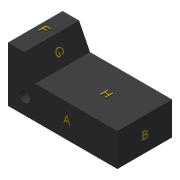
# Autodesk Inventor part: Component_1
Saved by Autodesk Inventor 2022 Beta2 (Build 260130000, 130) ContinuousBuild 0
## iProperties
Shininess: 64.0
Length Units: 11269
Angle Units: 11279
Time Units: 11290
Mass Units: 11283
Length Display Precision: 3
Angle Display Precision: 2
Compacted: True
Part Number: Component_1
Document SubType Name: Modeling
Created: 2004-04-20
Designer: mpaknia
Manufacturer: Standard
Standards Organization: Custom
Density: 1 g/cm^3
Material: Generic
Appearance: Generic
Density: 0.0
Volumn: 0.0
Area: 0.0
PropertySet Name: Model Information
Control State: 0
Master: False
Checked Out: False
Author: mpaknia
Autodesk Inventor part; units mm, degrees
note: some values were not read from the file. Chosen so that the rebuilt part matches the saved one: direction of "Emboss1"; direction of "Emboss2"; direction of "Emboss3"; direction of "Emboss4"; direction of "Emboss5".
ref_plane "YZ Plane" through (0, 0, 0) normal (1, 0, 0) x (0, 1, 0)
ref_plane "XZ Plane" through (0, 0, 0) normal (0, 1, 0) x (-1, 0, 0)
ref_plane "XY Plane" through (0, 0, 0) normal (0, 0, 1) x (1, 0, 0)
sketch "Sketch2" plane through (0, 0, 0) normal (0, 1, 0) x (-1, 0, 0)
  line L0 (0, 0) -> (100, 0)
  line L1 (100, 0) -> (100, 50)
  line L2 (100, 50) -> (85, 50)
  line L3 (85, 50) -> (75, 30)
  line L4 (75, 30) -> (0, 30)
  line L5 (0, 30) -> (0, 0)
  dimension "d5" = 100
  dimension "d6" = 50
  dimension "d7" = 30
  dimension "d8" = 15
  dimension "d9" = 75
  constraints: 12 end point, 3 parallel, 1 horizontal, 1 perpendicular
  measures "d5" distance of L0.start L0.end
  measures "d6" distance of L0.end L1.end
  measures "d7" distance of L4.end L0.start
  measures "d8" distance of L1.end L2.end
  measures "d9" distance of L3.end L4.end
extrude "Extrusion1" add sketch "Sketch2" along normal blind 50
sketch "Sketch3" plane through (0, 0, 0) normal (0, -1, 0) x (1, 0, 0)
  line L0 (0, 0) -> (-100, 0) projected
  line L1 (0, 30) -> (0, 0) projected
  point P0 (-85, 15)
  dimension "d12" = 85
  dimension "d13" = 15
  measures "d12" distance from line of L1 point (-85, 15)
  measures "d13" distance from line of L0 point (-85, 15)
hole "Hole1" at (-85, 0, 15) direction (0, 1, 0) diameter 10 end through all
sketch "Sketch4" plane through (0, 0, 0) normal (0, -1, 0) x (1, 0, 0)
  line L0 (-48.3615, 20.1685) -> (-41.8097, 20.1685) construction
  line L1 (-41.8097, 20.1685) -> (-41.8097, 13.1685) construction
  line L2 (-41.8097, 13.1685) -> (-48.3615, 13.1685) construction
  line L3 (-48.3615, 13.1685) -> (-48.3615, 20.1685) construction
  line L4 (-48.3722, 13.1685) -> (-45.6831, 20.1685)
  line L5 (-45.6831, 20.1685) -> (-44.6801, 20.1685)
  line L6 (-44.6801, 20.1685) -> (-41.8203, 13.1685)
  line L7 (-41.8203, 13.1685) -> (-42.8767, 13.1685)
  line L8 (-42.8767, 13.1685) -> (-43.6877, 15.2867)
  line L9 (-43.6877, 15.2867) -> (-46.6222, 15.2867)
  line L10 (-46.6222, 15.2867) -> (-47.3904, 13.1685)
  line L11 (-47.3904, 13.1685) -> (-48.3722, 13.1685)
  line L12 (-46.3554, 16.0389) -> (-43.9758, 16.0389)
  line L13 (-43.9758, 16.0389) -> (-44.7121, 17.981)
  spline S0 degree 2 poles (-44.7121, 17.981) (-45.0429, 18.8667) (-45.2029, 19.4322) knots 0 0 0 1 1 1
  spline S1 degree 2 poles (-45.2029, 19.4322) (-45.3417, 18.76) (-45.5818, 18.0931) knots 0 0 0 1 1 1
  line L14 (-45.5818, 18.0931) -> (-46.3554, 16.0389)
  constraints: 2 other
emboss "Emboss1" sketch "Sketch4" operation add depth 1 direction (0, 1, 0)
sketch "Sketch5" plane through (0, 0, 30) normal (1, 0, 0) x (0, 0, -1)
  line L0 (11.2488, 21.2339) -> (11.2488, 27.759) construction
  line L1 (11.2488, 27.759) -> (18.2488, 27.759) construction
  line L2 (18.2488, 27.759) -> (18.2488, 21.2339) construction
  line L3 (18.2488, 21.2339) -> (11.2488, 21.2339) construction
  line L4 (18.2488, 21.9488) -> (11.2488, 21.9488)
  line L5 (11.2488, 21.9488) -> (11.2488, 24.5738)
  spline S0 degree 4 poles (11.2488, 24.5738) (11.2488, 25.3741) (11.6756, 26.3451) (12.556, 26.8947) (13.0415, 26.8947) knots 0 0 0 0 0 1 1 1 1 1
  spline S1 degree 3 poles (13.0415, 26.8947) (13.4896, 26.8947) (14.2793, 26.4092) (14.5247, 25.913) knots 0 0 0 0 1 1 1 1
  spline S2 degree 3 poles (14.5247, 25.913) (14.7114, 26.5532) (15.6078, 27.2362) (16.2213, 27.2362) knots 0 0 0 0 1 1 1 1
  spline S3 degree 5 poles (16.2213, 27.2362) (16.7122, 27.2362) (17.5552, 26.82) (18.014, 26.2118) (18.2488, 25.2887) (18.2488, 24.6165) knots 0 0 0 0 0 0 1 1 1 1 1 1
  line L6 (18.2488, 24.6165) -> (18.2488, 21.9488)
  line L7 (17.4218, 22.8772) -> (17.4218, 24.6218)
  spline S4 degree 2 poles (17.4218, 24.6218) (17.4218, 25.07) (17.3898, 25.2514) knots 0 0 0 1 1 1
  spline S5 degree 4 poles (17.3898, 25.2514) (17.3311, 25.5715) (17.0643, 26.0037) (16.5521, 26.2811) (16.216, 26.2811) knots 0 0 0 0 0 1 1 1 1 1
  spline S6 degree 4 poles (16.216, 26.2811) (15.8265, 26.2811) (15.2503, 25.8703) (15.0156, 25.1607) (15.0156, 24.4938) knots 0 0 0 0 0 1 1 1 1 1
  line L8 (15.0156, 24.4938) -> (15.0156, 22.8772)
  line L9 (15.0156, 22.8772) -> (17.4218, 22.8772)
  line L10 (14.1886, 22.8772) -> (14.1886, 24.3871)
  spline S7 degree 2 poles (14.1886, 24.3871) (14.1886, 25.006) (14.1085, 25.2727) knots 0 0 0 1 1 1
  spline S8 degree 3 poles (14.1085, 25.2727) (14.0018, 25.6249) (13.5163, 25.9823) (13.1482, 25.9823) knots 0 0 0 0 1 1 1 1
  spline S9 degree 4 poles (13.1482, 25.9823) (12.8014, 25.9823) (12.2732, 25.6462) (12.0758, 25.0273) (12.0758, 24.275) knots 0 0 0 0 0 1 1 1 1 1
  line L11 (12.0758, 24.275) -> (12.0758, 22.8772)
  line L12 (12.0758, 22.8772) -> (14.1886, 22.8772)
  constraints: 2 other
emboss "Emboss2" sketch "Sketch5" operation add depth 1 direction (-1, 0, 0)
sketch "Sketch6" plane through (-75, 0, 30) normal (0, 0, 1) x (1, 0, 0)
  line L0 (37.9602, 27.186) -> (45.0242, 27.186) construction
  line L1 (45.0242, 27.186) -> (45.0242, 20.186) construction
  line L2 (45.0242, 20.186) -> (37.9602, 20.186) construction
  line L3 (37.9602, 20.186) -> (37.9602, 27.186) construction
  line L4 (38.7498, 20.186) -> (38.7498, 27.186)
  line L5 (38.7498, 27.186) -> (39.6782, 27.186)
  line L6 (39.6782, 27.186) -> (39.6782, 24.3102)
  line L7 (39.6782, 24.3102) -> (43.3062, 24.3102)
  line L8 (43.3062, 24.3102) -> (43.3062, 27.186)
  line L9 (43.3062, 27.186) -> (44.2346, 27.186)
  line L10 (44.2346, 27.186) -> (44.2346, 20.186)
  line L11 (44.2346, 20.186) -> (43.3062, 20.186)
  line L12 (43.3062, 20.186) -> (43.3062, 23.4833)
  line L13 (43.3062, 23.4833) -> (39.6782, 23.4833)
  line L14 (39.6782, 23.4833) -> (39.6782, 20.186)
  line L15 (39.6782, 20.186) -> (38.7498, 20.186)
  constraints: 2 other
emboss "Emboss3" sketch "Sketch6" operation add depth 1 direction (0, 0, -1)
sketch "Sketch7" plane through (-85, 0, 50) normal (0.8944272, 0, 0.4472136) x (0.4472136, 0, -0.8944272)
  line L0 (7.6622, 29.7722) -> (15.2704, 29.7722) construction
  line L1 (15.2704, 29.7722) -> (15.2704, 22.5321) construction
  line L2 (15.2704, 22.5321) -> (7.6622, 22.5321) construction
  line L3 (7.6622, 22.5321) -> (7.6622, 29.7722) construction
  line L4 (11.6957, 25.3919) -> (11.6957, 26.2188)
  line L5 (11.6957, 26.2188) -> (14.6569, 26.2188)
  line L6 (14.6569, 26.2188) -> (14.6569, 23.6258)
  spline S0 degree 3 poles (14.6569, 23.6258) (13.9739, 23.0816) (12.5227, 22.5321) (11.7598, 22.5321) knots 0 0 0 0 1 1 1 1
  spline S1 degree 4 poles (11.7598, 22.5321) (10.73, 22.5321) (9.0441, 23.4178) (8.1851, 25.0877) (8.1851, 26.1175) knots 0 0 0 0 0 1 1 1 1 1
  spline S2 degree 4 poles (8.1851, 26.1175) (8.1851, 27.1419) (9.0387, 28.9132) (10.6447, 29.7722) (11.6904, 29.7722) knots 0 0 0 0 0 1 1 1 1 1
  spline S3 degree 4 poles (11.6904, 29.7722) (12.448, 29.7722) (13.6751, 29.2813) (14.3687, 28.401) (14.5501, 27.6914) knots 0 0 0 0 0 1 1 1 1 1
  line L7 (14.5501, 27.6914) -> (13.7178, 27.462)
  spline S4 degree 4 poles (13.7178, 27.462) (13.5578, 27.9955) (13.0936, 28.6091) (12.2239, 28.9772) (11.6957, 28.9772) knots 0 0 0 0 0 1 1 1 1 1
  spline S5 degree 4 poles (11.6957, 28.9772) (11.0608, 28.9772) (10.1325, 28.5931) (9.5669, 27.9582) (9.4069, 27.5847) knots 0 0 0 0 0 1 1 1 1 1
  spline S6 degree 2 poles (9.4069, 27.5847) (9.1401, 26.9338) (9.1401, 26.1762) knots 0 0 0 1 1 1
  spline S7 degree 4 poles (9.1401, 26.1762) (9.1401, 25.2425) (9.7857, 23.978) (11.0181, 23.3698) (11.7064, 23.3698) knots 0 0 0 0 0 1 1 1 1 1
  spline S8 degree 3 poles (11.7064, 23.3698) (12.3093, 23.3698) (13.4564, 23.8339) (13.7498, 24.0954) knots 0 0 0 0 1 1 1 1
  line L8 (13.7498, 24.0954) -> (13.7498, 25.3919)
  line L9 (13.7498, 25.3919) -> (11.6957, 25.3919)
  constraints: 2 other
emboss "Emboss4" sketch "Sketch7" operation add depth 1 direction (-0.8944272, 0, -0.4472136)
sketch "Sketch8" plane through (-100, 0, 50) normal (0, 0, 1) x (1, 0, 0)
  line L0 (4.1672, 29.6786) -> (10.1428, 29.6786) construction
  line L1 (10.1428, 29.6786) -> (10.1428, 22.6786) construction
  line L2 (10.1428, 22.6786) -> (4.1672, 22.6786) construction
  line L3 (4.1672, 22.6786) -> (4.1672, 29.6786) construction
  line L4 (4.9675, 22.6786) -> (4.9675, 29.6786)
  line L5 (4.9675, 29.6786) -> (9.6946, 29.6786)
  line L6 (9.6946, 29.6786) -> (9.6946, 28.8516)
  line L7 (9.6946, 28.8516) -> (5.8959, 28.8516)
  line L8 (5.8959, 28.8516) -> (5.8959, 26.6854)
  line L9 (5.8959, 26.6854) -> (9.1825, 26.6854)
  line L10 (9.1825, 26.6854) -> (9.1825, 25.8584)
  line L11 (9.1825, 25.8584) -> (5.8959, 25.8584)
  line L12 (5.8959, 25.8584) -> (5.8959, 22.6786)
  line L13 (5.8959, 22.6786) -> (4.9675, 22.6786)
  constraints: 2 other
emboss "Emboss5" sketch "Sketch8" operation add depth 1 direction (0, 0, -1)
body "Solid1"
